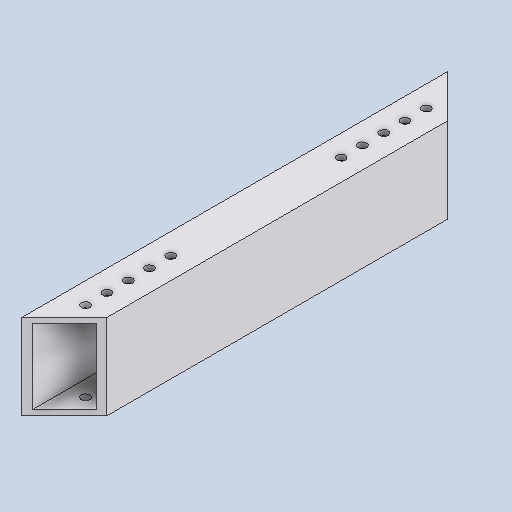
# Autodesk Inventor part: TUBE,ELEVATOR,BOT,STAGE1
Saved by Autodesk Inventor 2025.2 (Build 292293000, 293)
## iProperties
ILogicPurgeVersion: 0.0.0.0
Created: 2025-01-26
Part Number: TUBE,ELEVATOR,BOT,STAGE1
Material: Aluminum, 6063-T6
Document SubType Name: Modeling
Designer: Jthib
Density: 2.69879 g/cm^3
Appearance: Metal-AL-6063
Mass: 1095.07 g
Surface Area: 2563.7 cm^2
Volume: 405.58 cm^3
ModelCat: Uncategorized
Author: Jthib
Autodesk Inventor part; units mm, degrees
ref_plane "YZ Plane" through (0, 0, 0) normal (1, 0, 0) x (0, 1, 0)
ref_plane "XZ Plane" through (0, 0, 0) normal (0, 1, 0) x (-1, 0, 0)
ref_plane "XY Plane" through (0, 0, 0) normal (0, 0, 1) x (1, 0, 0)
sketch "Sketch1" plane through (0, 0, 0) normal (0, 0, 1) x (1, 0, 0)
  line L0 (-12.7, -25.4) -> (12.7, -25.4)
  line L1 (12.7, -25.4) -> (12.7, 25.4)
  line L2 (12.7, 25.4) -> (-12.7, 25.4)
  line L3 (-12.7, 25.4) -> (-12.7, -25.4)
  line L4 (-12.7, -25.4) -> (12.7, 25.4) construction
  line L5 (12.7, -25.4) -> (-12.7, 25.4) construction
  line L6 (-9.525, 22.225) -> (9.525, 22.225)
  line L7 (9.525, 22.225) -> (9.525, -22.225)
  line L8 (9.525, -22.225) -> (-9.525, -22.225)
  line L9 (-9.525, -22.225) -> (-9.525, 22.225)
  point P0 (0, 0)
  dimension "d0" = 25.4
  dimension "d1" = 50.8
  dimension "d2" = 3.175
  constraints: 20 end point, 4 parallel, 2 midpoint, 2 perpendicular, 1 horizontal, 3 other
  measures "d0" distance of L2.end L1.end
  measures "d1" distance of L1.end L0.end
  measures "d2" distance between parallel lines of L2 L6
extrude "Extrusion1" add sketch "Sketch1" along normal mid plane 254
sketch "Sketch2" plane through (-12.7, -25.4, 127) normal (0, -1, 0) x (1, 0, 0)
  line L0 (25.4, 0) -> (25.4, -254) projected
  line L1 (0, 0) -> (25.4, 0) construction
  line L2 (0, -254) -> (0, 0) construction
  line L3 (25.4, -254) -> (0, -254) projected
  line L4 (0, -254) -> (25.4, -228.6)
  point P0 (12.7, -127)
  dimension "d6" = 45
  constraints: 2 end point, 1 point on line
  measures "d6" angle of L2 L4
extrude "Extrusion2" cut sketch "Sketch2" against normal through all
sketch "Sketch4" plane through (-12.7, -25.4, 127) normal (0, -1, 0) x (1, 0, 0)
  line L0 (0, -254) -> (0, 0) construction
  point P0 (12.7, -127)
  point P1 (12.7, -228.6)
  point P2 (12.7, -215.9)
  point P3 (12.7, -203.2)
  point P4 (12.7, -190.5)
  point P5 (12.7, -177.8)
  dimension "d9" = 12.7
  dimension "d10" = 25.4
  dimension "d13" = 12.7
  constraints: 1 vertical, 4 other
  measures "d9" distance from line of L0 point (12.7, -228.6)
  measures "d10" vertical distance of L0.start point (12.7, -228.6)
  measures "d13" distance of point (12.7, -228.6) point (12.7, -215.9)
hole "Hole1" at (0, -25.4, -101.6) at (0, -25.4, -88.9) at (0, -25.4, -76.2) at (0, -25.4, -63.5) at (0, -25.4, -50.8) direction (0, 1, 0) diameter 5.1054 end through all start extended yes clearance for "Flat Head Machine Screw (82)" size "#10" standard "Ansi Unified Screw Threads"
mirror "Mirror1" about plane through (0, 0, 0) normal (0, 0, 1) of "Hole1", "Extrusion2"
body "Solid1"
